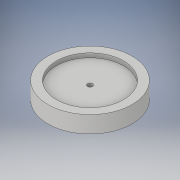
# Autodesk Inventor part: Rad
Saved by Autodesk Inventor 2019.5 (Build 235369000, 369)
## iProperties
Created: 2021-10-01
Part Number: Rad
Material: Generisch
Document SubType Name: Modeling
Designer: mritt
Density: 1 g/cm^3
Appearance: Vorgabe
Author: mritt
Autodesk Inventor part; units mm, degrees
ref_plane "YZ Plane" through (0, 0, 0) normal (1, 0, 0) x (0, 1, 0)
ref_plane "XZ Plane" through (0, 0, 0) normal (0, 1, 0) x (-1, 0, 0)
ref_plane "XY Plane" through (0, 0, 0) normal (0, 0, 1) x (1, 0, 0)
sketch "Skizze1" plane through (0, 0, 0) normal (0, 1, 0) x (-1, 0, 0)
  circle A0 centre (36.1244, -29.8236) radius 25
  circle A1 centre (36.1244, -29.8236) radius 1.5
  circle A2 centre (36.1244, -29.8236) radius 20
  point P0 (0, 0)
  dimension "d0" = 50
  dimension "d1" = 40
  dimension "d2" = 3
  constraints: 3 centre point, 2 coincident
  measures "d0" diameter of A0
  measures "d1" diameter of A2
  measures "d2" diameter of A1
extrude "Extrusion1" add sketch "Skizze1" along normal blind 5 and the other way blind 5 contours A0
extrude "Extrusion2" add sketch "Skizze1" along normal blind 2.5 and the other way blind 2.5 contours A2
